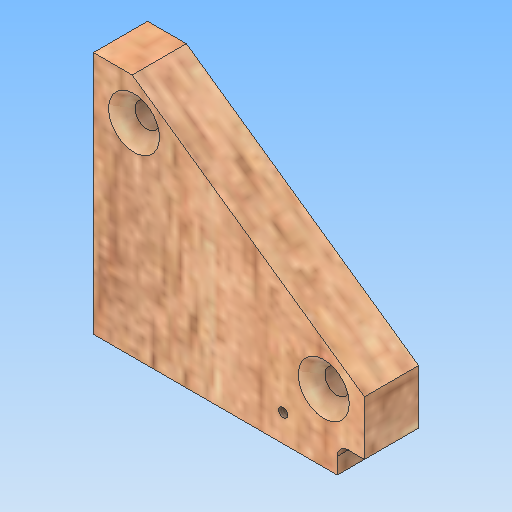
# Autodesk Inventor part: Pancake_Side Piece Short
Saved by Autodesk Inventor 2018.1 (Build 221171000, 171)
## iProperties
Created: 2019-02-21
Part Number: Pancake_Side Piece Short
Material: Wood (Birch)
Document SubType Name: Modeling
Designer: James
Density: 0.55 g/cm^3
Appearance: Birch - Natural Polished
Mass: 8.46056 g
Surface Area: 50.8226 cm^2
Volume: 15.3828 cm^3
Author: James
Autodesk Inventor part; units mm, degrees
ref_plane "YZ Plane" through (0, 0, 0) normal (1, 0, 0) x (0, 1, 0)
ref_plane "XZ Plane" through (0, 0, 0) normal (0, 1, 0) x (-1, 0, 0)
ref_plane "XY Plane" through (0, 0, 0) normal (0, 0, 1) x (1, 0, 0)
sketch "Sketch1" plane through (0, 0, 0) normal (0, 0, 1) x (1, 0, 0)
  line L0 (0, 0) -> (-50, 0)
  line L1 (-50, 40) -> (0, 40)
  line L2 (0, 40) -> (0, 0)
  line L3 (-50, 0) -> (-50, 40)
  line L4 (-50, 0) -> (-5, 0)
  line L5 (-5, 0) -> (-5, -5)
  line L6 (-5, -5) -> (-50, -5)
  line L7 (-50, -5) -> (-50, 0)
  dimension "d1" = 40
  dimension "d2" = 50
  dimension "d20" = 5
  dimension "d21" = 5
  constraints: 16 end point, 3 parallel, 2 horizontal, 2 vertical, 1 perpendicular
  measures "d1" distance of L1.end L0.start
  measures "d2" distance of L0.start L0.end
  measures "d20" distance between parallel lines of L2 L5
  measures "d21" distance of L4.end L5.end
extrude "Extrusion1" add sketch "Sketch1" along normal blind 10
sketch "Sketch2" plane through (0, 0, 10) normal (0, 0, 1) x (1, 0, 0)
  line L0 (0, 40) -> (-50, 40) projected
  line L1 (0, 0) -> (0, 40) projected
  line L2 (-5, 0) -> (0, 0) projected
  line L3 (-50, 40) -> (-50, -5) projected
  point P0 (-42.5, 32.5)
  point P1 (-7.5, 7.5)
  point P2 (-50, 0)
  dimension "d5" = 7.5
  dimension "d7" = 7.5
  dimension "d15" = 7.5
  dimension "d16" = 7.5
  measures "d5" distance from line of point (-42.5, 32.5) L0
  measures "d7" distance from line of L2 point (-7.5, 7.5)
  measures "d15" distance from line of point (-42.5, 32.5) L3
  measures "d16" distance from line of L1 point (-7.5, 7.5)
hole "Hole1" at (-42.5, 32.5, 10) at (-7.5, 7.5, 10) direction (0, 0, -1) diameter 4.5 end through all countersink diameter 9.4 countersink angle 90 clearance for "Flat Head Machine Screw" size "M4" standard "Ansi Metric M Profile"
chamfer "Chamfer1" distance 30 angle 55 1 edges at (0, 40, 5) measured on face at (0, 26.6667, 3.3333)
fillet "Fillet1" radius 2 1 edges at (-5, 0, 5)
sketch "Sketch3" plane through (0, 0, 10) normal (0, 0, 1) x (1, 0, 0)
  line L0 (-50, -5) -> (-5, -5) projected
  line L1 (0, 0) -> (0, 10) projected
  point P0 (-15, 0)
  dimension "d23" = 5
  dimension "d24" = 15
  measures "d23" distance from line of point (-15, 0) L0
  measures "d24" distance from line of L1 point (-15, 0)
hole "Hole2" at (-15, 0, 10) direction (0, 0, -1) diameter 1.694 depth 6.637 tip angle 118 thread size "2-56 UNC" class "2B" standard "ANSI Unified Screw Threads"
equation "\"d7\" = d5"
equation "\"d15\" = d16"
body "Solid1"
